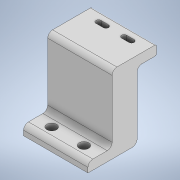
# Autodesk Inventor part: MagnetActuatorHolder
Saved by Autodesk Inventor 2021 (Build 250183000, 183)
## iProperties
Created: 2021-12-05
Part Number: MagnetActuatorHolder
Material: Generic
Document SubType Name: Modeling
Designer: Jorian Brusind
Density: 1 g/cm^3
Appearance: Default
Author: Jorian Brusind
Autodesk Inventor part; units mm, degrees
ref_plane "YZ Plane" through (0, 0, 0) normal (1, 0, 0) x (0, 1, 0)
ref_plane "XZ Plane" through (0, 0, 0) normal (0, 1, 0) x (-1, 0, 0)
ref_plane "XY Plane" through (0, 0, 0) normal (0, 0, 1) x (1, 0, 0)
sketch "Sketch1" plane through (0, 0, 0) normal (0, 1, 0) x (-1, 0, 0)
  line L0 (0, 0) -> (34, 0)
  line L1 (34, 0) -> (34, -9.53)
  line L2 (34, -9.53) -> (0, -9.53)
  line L3 (0, -9.53) -> (0, 0)
  line L4 (37, -12.53) -> (37, 3)
  line L5 (37, 3) -> (-3, 3)
  line L6 (-3, 3) -> (-3, -12.53)
  line L7 (-3, -12.53) -> (37, -12.53)
  dimension "d0" = 34
  dimension "d1" = 9.53
  dimension "d2" = 3
  constraints: 16 end point, 4 parallel, 2 perpendicular, 1 horizontal, 3 other
  measures "d0" distance of L1.end L2.end
  measures "d1" distance of L0.end L1.end
  measures "d2" distance between parallel lines of L1 L4
extrude "Extrusion1" add sketch "Sketch1" along normal blind 48 contours L0 L1 L2 L3 | L7 L6 L5 L4
sketch "Sketch3" plane through (0, 0, 0) normal (0, -1, 0) x (1, 0, 0)
  line L0 (-37, 3) -> (3, 3) projected
  line L1 (-37, 3) -> (3, 3)
  line L2 (3, 3) -> (3, 18)
  line L3 (3, 18) -> (-37, 18)
  line L4 (-37, 18) -> (-37, 3)
  line L5 (3, -12.53) -> (-37, -12.53) projected
  line L6 (-37, -12.53) -> (3, -12.53)
  line L7 (3, -12.53) -> (3, -27.53)
  line L8 (3, -27.53) -> (-37, -27.53)
  line L9 (-37, -27.53) -> (-37, -12.53)
  circle A0 centre (-27, -20.03) radius 3
  circle A1 centre (-27, 10.5) radius 3
  circle A2 centre (-7, -20.03) radius 3
  circle A3 centre (-7, 10.5) radius 3
  point P0 (0, 0)
  dimension "d5" = 40
  dimension "d6" = 15
  dimension "d7" = 40
  dimension "d8" = 15
  dimension "d9" = 6
  dimension "d10" = 10
  dimension "d11" = 7.5
  dimension "d14" = 30.53
  dimension "d17" = 20
  constraints: 16 end point, 4 centre point, 4 parallel, 3 horizontal, 2 perpendicular, 1 vertical, 6 other
  measures "d5" distance of L3.end L2.end
  measures "d6" distance of L2.end L1.end
  measures "d7" distance of L7.end L8.end
  measures "d8" distance of L6.end L7.end
  measures "d9" diameter of A0
  measures "d10" distance from line of L9 A0.centre
  measures "d11" distance from line of L8 A0.centre
  measures "d14" distance of A0.centre A1.centre
  measures "d17" distance of A0.centre A2.centre
extrude "Extrusion2" add sketch "Sketch3" against normal blind 6 contours L4 L3 L2 L0
sketch "Sketch5" plane through (0, 48, 0) normal (0, 1, 0) x (1, 0, 0)
  line L0 (3, 12.53) -> (-37, 12.53) projected
  line L1 (-37, 12.53) -> (3, 12.53)
  line L2 (3, 12.53) -> (3, 24.53)
  line L3 (3, 24.53) -> (-37, 24.53)
  line L4 (-37, 24.53) -> (-37, 12.53)
  line L5 (-37, 18.53) -> (-27, 18.53)
  line L6 (-27, 18.53) -> (-22.36, 18.53) construction
  line L7 (-27, 16.94) -> (-22.36, 16.94)
  line L8 (-22.36, 20.12) -> (-27, 20.12)
  arc A0 (-27, 20.12) -> (-27, 16.94) centre (-27, 18.53) ccw
  arc A1 (-22.36, 16.94) -> (-22.36, 20.12) centre (-22.36, 18.53) ccw
  line L9 (-27, 18.53) -> (-22.36, 18.53) construction
  line L10 (-22.36, 18.53) -> (-11.12, 18.53)
  line L11 (-22.36, 18.53) -> (-11.12, 18.53) construction
  line L12 (-11.12, 18.53) -> (-6.48, 18.53) construction
  line L13 (-11.12, 16.94) -> (-6.48, 16.94)
  line L14 (-6.48, 20.12) -> (-11.12, 20.12)
  arc A2 (-11.12, 20.12) -> (-11.12, 16.94) centre (-11.12, 18.53) ccw
  arc A3 (-6.48, 16.94) -> (-6.48, 20.12) centre (-6.48, 18.53) ccw
  point P0 (0, 0)
  point P1 (-24.68, 18.53)
  point P2 (-8.8, 18.53)
  dimension "d40" = 40
  dimension "d41" = 12
  dimension "d42" = 10
  dimension "d43" = 4.64
  dimension "d44" = 0
  dimension "d45" = 3.18
  dimension "d46" = 11.24
  dimension "d47" = 0
  dimension "d48" = 4.64
  dimension "d49" = 3.18
  constraints: 32 end point, 8 point on circle, 8 tangent, 7 horizontal, 4 centre point, 4 parallel, 3 midpoint, 2 collinear, 1 perpendicular
  measures "d40" distance of L3.end L2.end
  measures "d41" distance of L2.end L1.end
  measures "d42" distance of L5.start L5.end
  measures "d43" distance of L5.end L6.end
  measures "d44" distance between parallel lines of L6 L9
  measures "d45" diameter of A1
  measures "d46" distance of L9.end L10.end
  measures "d47" distance between parallel lines of L10 L11
  measures "d48" distance of L11.end L12.end
  measures "d49" diameter of A3
extrude "Extrusion4" add sketch "Sketch5" against normal blind 6
fillet "Fillet1" radius 3 1 edges at (-17, 42, -12.53)
fillet "Fillet2" radius 3 2 edges at (-17, 48, 3) (-17, 6, 3)
fillet "Fillet3" radius 3 1 edges at (-17, 6, 18)
fillet "Fillet4" radius 3 1 edges at (-17, 0, -12.53)
fillet "Fillet5" radius 1 2 edges at (-17, 48, -24.53) (-17, 42, -24.53)
body "Solid1"
